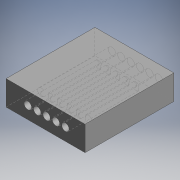
# Autodesk Inventor part: 00001_Single_Mode_Pan
Saved by Autodesk Inventor 2019 (Build 230136000, 136)
## iProperties
Part Number: 00001_Single_Mode_Pan
Material: Generic
Document SubType Name: Modeling
Designer: oriani
Appearance: Default
Author: oriani
Autodesk Inventor part; units mm, degrees
ref_plane "YZ Plane" through (0, 0, 0) normal (1, 0, 0) x (0, 1, 0)
ref_plane "XZ Plane" through (0, 0, 0) normal (0, 1, 0) x (-1, 0, 0)
ref_plane "XY Plane" through (0, 0, 0) normal (0, 0, 1) x (1, 0, 0)
sketch "Sketch1" plane through (0, 0, 0) normal (0, 0, 1) x (1, 0, 0)
  line L0 (0, 0) -> (-50.8, 0)
  line L1 (-50.8, 0) -> (-50.8, 15.875)
  line L2 (-50.8, 15.875) -> (0, 15.875)
  line L3 (0, 15.875) -> (0, 0)
  point P0 (-9.6497, 7.9375)
  point P1 (-15.6822, 7.9375)
  point P2 (-21.7147, 7.9375)
  point P3 (-27.7472, 7.9375)
  point P4 (-33.7797, 7.9375)
  point P5 (-39.8122, 7.9375)
  constraints: 8 end point
sketch "Sketch2" plane through (0, 0, 57.15) normal (0, 0, 1) x (1, 0, 0)
  point P0 (-12.666, 7.9375)
  point P1 (-18.6985, 7.9375)
  point P2 (-24.731, 7.9375)
  point P3 (-30.7635, 7.9375)
  point P4 (-36.796, 7.9375)
extrude "Extrusion1" add sketch "Sketch1" along normal blind 57.15
hole "Hole1" at (-9.6497, 7.9375, 0) at (-15.6822, 7.9375, 0) at (-21.7147, 7.9375, 0) at (-27.7472, 7.9375, 0) at (-33.7797, 7.9375, 0) at (-39.8122, 7.9375, 0) direction (0, 0, 1) diameter 4.7625 depth 45.4453 tip angle 118
hole "Hole2" at (-12.666, 7.9375, 57.15) at (-18.6985, 7.9375, 57.15) at (-24.731, 7.9375, 57.15) at (-30.7635, 7.9375, 57.15) at (-36.796, 7.9375, 57.15) direction (0, 0, -1) diameter 4.7625 depth 45.4453 tip angle 118
body "Solid1"
